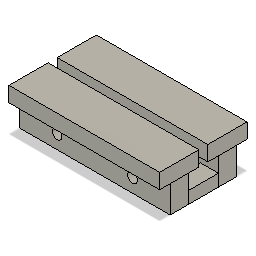
Bed v1 (Autodesk Fusion 360 design; units mm, degrees)
Autodesk Fusion 360 part; units mm, degrees
note: some values were not read from the file. Set by a fixed rule: which sketch regions a step uses.
sketch "Sketch1" plane through (0, 0, 0) normal (1, 0, 0) x (0, 0, -1) in component "Bottom"
  line L0 (-50, 0) -> (-110, 0)
  line L1 (-110, 0) -> (-110, 90)
  line L2 (-110, 90) -> (-50, 90)
  line L3 (-50, 90) -> (-50, 0)
  dimension "d1" = 60
  dimension "d2" = 90
  dimension "d3" = 50
  measures "d1" distance of origin
extrude "Extrude1" add sketch "Sketch1" along normal mid plane 500 makes body 1 in component "Bottom"
mirror "Mirror1" about plane through (0, 0, 0) normal (0, 0, 1) of bodies 1 makes body 2 in component "Bottom"
sketch "Sketch1 (2)" plane through (0, 0, 0) normal (1, 0, 0) x (0, 0, -1) in component "Flat"
  line L0 (-110, 90) -> (-50, 90)
  line L1 (-145, 90) -> (-15, 90)
  line L2 (-15, 90) -> (-15, 140)
  line L3 (-15, 140) -> (-145, 140)
  line L4 (-145, 140) -> (-145, 90)
  dimension "d7" = 130
  dimension "d8" = 50
  measures "d7" distance of origin
extrude "Extrude1'" add sketch "Sketch1 (2)" along normal mid plane 500 separate body makes body 3 in component "Flat"
mirror "Mirror1'" about plane through (0, 0, 0) normal (0, 0, 1) of bodies 3 makes body 4 in component "Flat"
sketch "Sketch1 (3)" plane through (250, 0, 0) normal (1, 0, 0) x (0, 0, -1) in component "Spacers"
  line L0 (-50, 90) -> (-110, 90)
  line L1 (-110, 90) -> (-110, 0)
  line L2 (-110, 0) -> (-50, 0)
  line L3 (-50, 0) -> (-50, 90)
  line L4 (-50, 0) -> (-50, 90)
  line L5 (50, 0) -> (50, 90)
  line L6 (-50, 0) -> (50, 0)
  line L7 (50, 0) -> (50, 40)
  line L8 (50, 40) -> (-50, 40)
  line L9 (-50, 40) -> (-50, 0)
extrude "Extrude1''" add sketch "Sketch1 (3)" against normal blind 60 separate body contours L3 L4 L5 L6 L7 L8 L9 makes body 5 in component "Spacers"
mirror "Mirror1''" about plane through (0, 0, 0) normal (1, 0, 0) of bodies 5 makes body 6 in component "Spacers"
sketch "Sketch2" plane through (0, 0, 0) normal (0, 0, 1) x (1, 0, 0) in component "Bottom"
  line L0 (-250, 0) -> (250, 0)
  line L1 (250, 0) -> (250, 90)
  line L2 (250, 90) -> (-250, 90)
  line L3 (-250, 90) -> (-250, 0)
  line L4 (250, 90) -> (0, 0)
  line L5 (250, 0) -> (0, 90)
  line L6 (-250, 90) -> (0, 0)
  line L7 (-250, 0) -> (0, 90)
  circle A0 centre (125, 45) radius 16
  circle A1 centre (-125, 45) radius 16
  dimension "d15" = 32
  dimension "d16" = 32
  measures "d15" diameter of A0
  measures "d16" diameter of A1
extrude "Extrude2" cut sketch "Sketch2" along normal through all and the other way through all contours L6 L7 A1 | L6 L7 A1 | L4 L5 A0 | L4 L5 A0 | L6 L7 A1 | L6 L7 A1 | L4 L5 A0 | L4 L5 A0 bodies 1 2 in component "Bottom"
component "Bed" placed x (1, 0, 0) y (0, 1, 0) z (0, 0, 1) at (0, 0, 0)
component "Bottom" placed x (1, 0, 0) y (0, 1, 0) z (0, 0, 1) at (0, 0, 0) in component "Bed"
component "Flat" placed x (1, 0, 0) y (0, 1, 0) z (0, 0, 1) at (0, 0, 0) in component "Bed"
component "Spacers" placed x (1, 0, 0) y (0, 1, 0) z (0, 0, 1) at (0, 0, 0) in component "Bed"
